makerbeam-8cm-handle v2 (Autodesk Fusion 360 design; units mm, degrees)
Autodesk Fusion 360 part; units mm, degrees
box "BoxPrimitive1" add length 60 width 120 height 14 placed x (0, 0, -1) y (-1, 0, 0) z (0, 1, 0) at (120, 0, 0)
fillet "Fillet1" radius 20 1 edges at (0, 7, -60)
fillet "Fillet1" radius 20 1 edges at (120, 7, -60)
box "BoxPrimitive2" cut length 10 width 10 height -120 placed x (0, 1, 0) y (0, 0, 1) z (1, 0, 0) at (120, 2, -10)
box "BoxPrimitive3" cut length 30 width 80 height -60 placed x (0, 0, -1) y (-1, 0, 0) z (0, 1, 0) at (100, 14, -20)
fillet "Fillet2" radius 8 1 edges at (20, 7, -50)
fillet "Fillet2" radius 8 1 edges at (100, 7, -50)
fillet "Fillet2" radius 8 1 edges at (100, 7, -20)
fillet "Fillet2" radius 8 1 edges at (20, 7, -20)
cylinder "CylinderPrimitive1" cut diameter 3.1 height -15 placed x (1, 0, 0) y (0, 0, -1) z (0, 1, 0) at (60, 14, -5)
cylinder "CylinderPrimitive2" cut diameter 3.1 height -15 placed x (1, 0, 0) y (0, 0, -1) z (0, 1, 0) at (20, 14, -5)
cylinder "CylinderPrimitive3" cut diameter 3.1 height -15 placed x (1, 0, 0) y (0, 0, -1) z (0, 1, 0) at (100, 14, -5)
